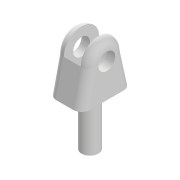
# Autodesk Inventor part: wrist
Saved by Autodesk Inventor 2020.2 (Build 242310000, 310)
## iProperties
Created: 2020-04-11
Part Number: wrist
Material: Generic
Document SubType Name: Modeling
Designer: Bardo91
Density: 1 g/cm^3
Appearance: Default
Author: Bardo91
Autodesk Inventor part; units mm, degrees
ref_plane "YZ Plane" through (0, 0, 0) normal (1, 0, 0) x (0, 1, 0)
ref_plane "XZ Plane" through (0, 0, 0) normal (0, 1, 0) x (-1, 0, 0)
ref_plane "XY Plane" through (0, 0, 0) normal (0, 0, 1) x (1, 0, 0)
sketch "Sketch1" plane through (0, 0, 0) normal (1, 0, 0) x (0, 1, 0)
  circle A0 centre (0, 0) radius 5
  circle A1 centre (0, 0) radius 10.5
  line L0 (0, 0) -> (-20, 0)
  line L1 (-20, 0) -> (-20, -15)
  line L2 (-20, -15) -> (-20, 15)
  line L3 (-20, 15) -> (0, 10.5)
  line L4 (0, -10.5) -> (-20, -15)
  dimension "d0" = 10
  dimension "d1" = 21
  dimension "d2" = 20
  dimension "d3" = 15
  dimension "d4" = 30
  constraints: 10 end point, 2 centre point, 2 coincident, 2 point on circle, 1 horizontal, 1 perpendicular, 1 point on line
  measures "d0" diameter of A0
  measures "d1" diameter of A1
  measures "d2" distance of L0.start L0.end
  measures "d3" distance of L0.end L1.end
  measures "d4" distance of L1.end L2.end
extrude "Extrusion1" add sketch "Sketch1" along normal blind 5
sketch "Sketch2" plane through (5, 0, 0) normal (1, 0, 0) x (0, 0, -1)
  arc A0 (10.5, 0) -> (-10.5, 0) centre (0, 0) ccw projected
  circle A1 centre (0, 0) radius 10.5
  line L0 (-10.5, 0) -> (-15, -20) projected
  line L1 (-10.5, 0) -> (-15, -20)
  line L2 (15, -20) -> (10.5, 0) projected
  line L3 (-15, -20) -> (15, -20)
  line L4 (15, -20) -> (10.5, 0)
  point P0 (-10.5, 0)
  constraints: 6 end point, 2 point on circle, 1 centre point, 1 coincident, 1 collinear, 1 horizontal, 1 point on line
extrude "Extrusion2" add sketch "Sketch2" along normal blind 10 contours L2 L3 L0 A1
sketch "Sketch4" plane through (15, 0, 0) normal (1, 0, 0) x (0, 0, -1)
  circle A0 centre (0, 0) radius 5
  circle A1 centre (0, 0) radius 10.5
  line L0 (15, -20) -> (10.5, 0) projected
  line L1 (10.5, 0) -> (15, -20)
  line L2 (-15, -20) -> (15, -20) projected
  line L3 (15, -20) -> (-15, -20)
  line L4 (-10.5, 0) -> (-15, -20) projected
  line L5 (-15, -20) -> (-10.5, 0)
  constraints: 6 end point, 3 collinear, 2 centre point, 2 coincident, 1 point on circle
extrude "Extrusion3" add sketch "Sketch4" along normal blind 5
sketch "Sketch5" plane through (0, -20, -15) normal (0, -1, 0) x (1, 0, 0)
  line L0 (20, 4.5) -> (20, 25.5) projected
  line L1 (20, 15) -> (0, 15)
  circle A0 centre (10, 15) radius 5
  dimension "d11" = 10
  constraints: 2 end point, 2 midpoint, 1 centre point, 1 horizontal
  measures "d11" diameter of A0
extrude "Extrusion4" add sketch "Sketch5" along normal blind 30
fillet "Fillet1" radius 5 6 edges at (20, -10, 12.75) (20, -10, -12.75) (20, 10.5, 0) (0, 10.5, 0) (0, -10, -12.75) (0, -10, 12.75)
body "Solid1"
